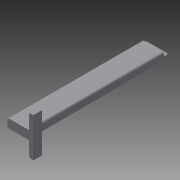
# Autodesk Inventor part: Main Stand
Saved by Autodesk Inventor 2015 (Build 190159000, 159)
## iProperties
Created: 2016-05-27
Part Number: Main Stand
Material: Generic
Document SubType Name: Modeling
Designer: Toby
Density: 1 g/cm^3
Appearance: Default
Author: Toby
Autodesk Inventor part; units mm, degrees
ref_plane "YZ Plane" through (0, 0, 0) normal (1, 0, 0) x (0, 1, 0)
ref_plane "XZ Plane" through (0, 0, 0) normal (0, 1, 0) x (-1, 0, 0)
ref_plane "XY Plane" through (0, 0, 0) normal (0, 0, 1) x (1, 0, 0)
sketch "Sketch1" plane through (0, 0, 0) normal (0, 1, 0) x (-1, 0, 0)
  line L0 (1.4527, 22.4324) -> (-3.5473, 22.4324)
  line L1 (-3.5473, 22.4324) -> (-3.5473, -22.5676)
  line L2 (-3.5473, -22.5676) -> (1.4527, -22.5676)
  line L3 (1.4527, -22.5676) -> (1.4527, 22.4324)
  line L4 (-3.5473, 4.9324) -> (26.4527, 4.9324)
  line L5 (26.4527, 4.9324) -> (26.4527, -5.0676)
  line L6 (26.4527, -5.0676) -> (-3.5473, -5.0676)
  line L7 (-3.5473, -5.0676) -> (-3.5473, 4.9324)
  point P0 (0, 0)
  dimension "d0" = 45
  dimension "d1" = 30
  dimension "d2" = 10
  dimension "d3" = 17.5
  dimension "d4" = 17.5
  dimension "d5" = 5
  constraints: 16 end point, 4 parallel, 2 horizontal, 2 perpendicular, 1 point on line
  measures "d0" distance of L0.end L1.end
  measures "d1" distance of L5.end L6.end
  measures "d2" distance of L4.end L5.end
  measures "d3" distance between parallel lines of L0 L4
  measures "d4" distance between parallel lines of L6 L2
  measures "d5" distance of L0.start L0.end
extrude "Extrusion1" add sketch "Sketch1" along normal blind 10
sketch "Sketch2" plane through (0, 10, 0) normal (0, 1, 0) x (1, 0, 0)
  line L0 (-26.4527, -4.9324) -> (-1.4527, -4.9324)
  line L1 (-1.4527, -4.9324) -> (-1.4527, 5.0676)
  line L2 (-1.4527, 5.0676) -> (-26.4527, 5.0676)
  line L3 (-26.4527, 5.0676) -> (-26.4527, -4.9324)
  point P0 (0, 0)
  constraints: 8 end point, 2 parallel, 1 horizontal, 1 perpendicular
extrude "Extrusion2" add sketch "Sketch2" along normal blind 145
fillet "Fillet1" radius 2 1 edges at (-1.4527, 10, -0.0676)
sketch "Sketch3" plane through (0, 155, 0) normal (0, 1, 0) x (1, 0, 0)
  line L0 (-26.4527, 5.0676) -> (-26.4527, -4.9324) projected
  line L1 (-1.4527, 5.0676) -> (-1.4527, -4.9324) projected
  line L2 (-26.4527, -0.9324) -> (-1.4527, -0.9324)
  line L3 (-1.4527, -0.9324) -> (-1.4527, 1.0676)
  line L4 (-1.4527, 1.0676) -> (-26.4527, 1.0676)
  line L5 (-26.4527, 1.0676) -> (-26.4527, -0.9324)
  line L6 (-26.4527, -4.9324) -> (-1.4527, -4.9324) projected
  line L7 (-1.4527, 5.0676) -> (-26.4527, 5.0676) projected
  point P0 (0, 0)
  dimension "d11" = 2
  dimension "d12" = 4
  dimension "d13" = 4
  constraints: 8 end point, 2 parallel, 2 point on line, 1 horizontal, 1 perpendicular
  measures "d11" distance between parallel lines of L4 L2
  measures "d12" distance between parallel lines of L6 L2
  measures "d13" distance between parallel lines of L7 L4
extrude "Extrusion3" add sketch "Sketch3" along normal blind 5 contours L4 L1 L2 L0
fillet "Fillet2" radius 2 6 edges at (-0.8669, 10.5858, 4.9324) (-1.4527, 83.5, 4.9324) (-0.8669, 10.5858, -5.0676) (-1.4527, 83.5, -5.0676) (-26.4527, 77.5, -5.0676) (-26.4527, 77.5, 4.9324)
fillet "Fillet3" radius 2 2 edges at (-1.4527, 5, 22.4324) (-1.4527, 5, -22.5676)
body "Solid1"
